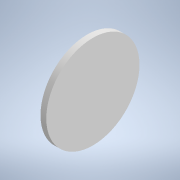
# Autodesk Inventor part: тест2
Saved by Autodesk Inventor 2022 (Build 260153070, 153G)
## iProperties
Created: 2021-09-16
Part Number: тест2
Material: Типовые
Document SubType Name: Modeling
Designer: Алексанян Г.
Density: 1 g/cm^3
Appearance: По умолчанию
Author: Алексанян Г.
Autodesk Inventor part; units mm, degrees
ref_plane "YZ Plane" through (0, 0, 0) normal (1, 0, 0) x (0, 1, 0)
ref_plane "XZ Plane" through (0, 0, 0) normal (0, 1, 0) x (-1, 0, 0)
ref_plane "XY Plane" through (0, 0, 0) normal (0, 0, 1) x (1, 0, 0)
sketch "Эскиз1" plane through (0, 0, 0) normal (1, 0, 0) x (0, 1, 0)
  circle A0 centre (105.9487, 80.6132) radius 81.2133
  point P0 (0, 0)
  dimension "d0" = 10
  constraints: 1 centre point
extrude "Выдавливание1" add sketch "Эскиз1" along normal blind 10
